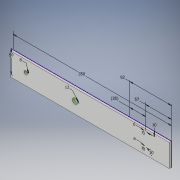
# Autodesk Inventor part: OldalsoSzuport
Saved by Autodesk Inventor 2019 (Build 230136000, 136)
## iProperties
Created: 2022-08-26
Part Number: OldalsoSzuport
Material: Generic
Document SubType Name: Modeling
Designer: laca
Density: 1 g/cm^3
Appearance: Default
Author: laca
Autodesk Inventor part; units mm, degrees
ref_plane "YZ Plane" through (0, 0, 0) normal (1, 0, 0) x (0, 1, 0)
ref_plane "XZ Plane" through (0, 0, 0) normal (0, 1, 0) x (-1, 0, 0)
ref_plane "XY Plane" through (0, 0, 0) normal (0, 0, 1) x (1, 0, 0)
sketch "Sketch1" plane through (0, 0, 0) normal (0, 0, 1) x (1, 0, 0)
  line L0 (0, 0) -> (-350, 0)
  line L1 (-350, 0) -> (-350, 50)
  line L2 (-350, 50) -> (0, 50)
  line L3 (0, 50) -> (0, 0)
  circle A0 centre (-57, 40) radius 3
  circle A1 centre (-57, 10) radius 3
  line L4 (-92, 50) -> (-92, 18.4785)
  circle A2 centre (-208.0745, 25) radius 6
  circle A3 centre (-316.9122, 25) radius 4
  dimension "d0" = 350
  dimension "d1" = 50
  dimension "d2" = 6
  dimension "d3" = 6
  dimension "d4" = 10
  dimension "d5" = 10
  dimension "d6" = 57
  dimension "d7" = 92
  dimension "d8" = 35
  dimension "d11" = 12
  dimension "d12" = 8
  constraints: 10 end point, 4 centre point, 2 parallel, 1 horizontal, 1 perpendicular, 1 point on line, 1 vertical, 1 vertical alignment
  measures "d0" distance of L1.end L2.end
  measures "d1" distance of L0.end L1.end
  measures "d2" diameter of A0
  measures "d3" diameter of A1
  measures "d4" distance from line of L2 A0.centre
  measures "d5" distance from line of L0 A1.centre
  measures "d6" distance from line of L3 A0.centre
  measures "d7" distance between parallel lines of L3 L4
  measures "d8" distance from line of L4 A0.centre
  measures "d11" diameter of A2
  measures "d12" diameter of A3
extrude "Extrusion1" add sketch "Sketch1" along normal blind 5 contours L0 L1 L2 L3 | A2 | A3
extrude "Extrusion2" cut sketch "Sketch1" along normal through all contours A2 | A3
body "Solid1"
